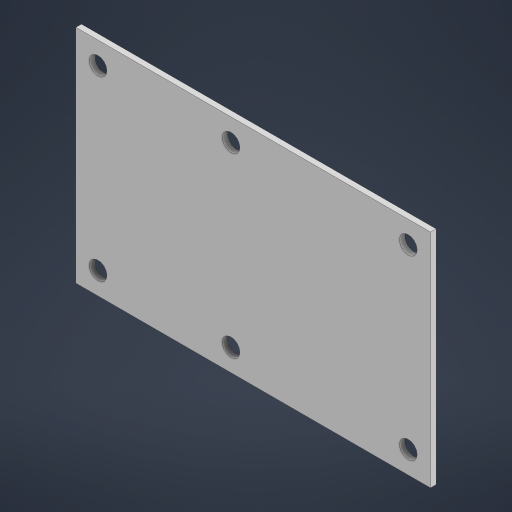
# Autodesk Inventor part: kickPlate
Saved by Autodesk Inventor 2023.4 (Build 274418000, 418)
## iProperties
Created: 2024-01-28
Part Number: kickPlate
Material: Generic
Document SubType Name: Modeling
Designer: Meer
Density: 1 g/cm^3
Appearance: Default
Author: Meer
Autodesk Inventor part; units mm, degrees
ref_plane "YZ Plane" through (0, 0, 0) normal (1, 0, 0) x (0, 1, 0)
ref_plane "XZ Plane" through (0, 0, 0) normal (0, 1, 0) x (-1, 0, 0)
ref_plane "XY Plane" through (0, 0, 0) normal (0, 0, 1) x (1, 0, 0)
sketch "Sketch1" plane through (0, 0, 0) normal (0, 0, 1) x (1, 0, 0)
  line L0 (0, 0) -> (101.6, 0)
  line L1 (101.6, 0) -> (101.6, 63.5)
  line L2 (101.6, 63.5) -> (0, 63.5)
  line L3 (0, 63.5) -> (0, 0)
  line L4 (7.1778, 63.5) -> (7.1778, 57.15)
  line L5 (0, 57.15) -> (6.35, 57.15)
  line L6 (6.35, 57.15) -> (44.45, 57.15)
  line L7 (44.45, 57.15) -> (95.25, 57.15)
  circle A0 centre (44.45, 57.15) radius 2.54
  circle A1 centre (95.25, 57.15) radius 2.54
  circle A2 centre (6.35, 57.15) radius 2.54
  line L8 (6.35, 0) -> (6.35, 6.35)
  line L9 (0, 6.35) -> (6.35, 6.35)
  line L10 (6.35, 6.35) -> (44.45, 6.35)
  line L11 (44.45, 6.35) -> (69.85, 6.35)
  line L12 (69.85, 6.35) -> (95.25, 6.35)
  circle A3 centre (6.35, 6.35) radius 2.54
  circle A4 centre (44.45, 6.35) radius 2.54
  circle A5 centre (95.25, 6.35) radius 2.54
  dimension "d0" = 101.6
  dimension "d1" = 63.5
  dimension "d2" = 6.35
  dimension "d3" = 6.35
  dimension "d5" = 38.1
  dimension "d6" = 50.8
  dimension "d7" = 5.08
  dimension "d8" = 5.08
  dimension "d9" = 5.08
  dimension "d12" = 6.35
  dimension "d13" = 6.35
  dimension "d14" = 38.1
  dimension "d15" = 25.4
  dimension "d16" = 25.4
  dimension "d17" = 5.08
  dimension "d18" = 5.08
  dimension "d19" = 5.08
  constraints: 26 end point, 8 point on line, 7 coincident, 6 centre point, 4 perpendicular, 3 parallel, 2 horizontal
  measures "d0" distance of L2.end L1.end
  measures "d1" distance of L1.end L0.end
  measures "d2" distance of L4.start L4.end
  measures "d3" distance of L5.start L5.end
  measures "d5" distance of L6.start L6.end
  measures "d6" distance of L6.end L7.end
  measures "d7" diameter of A0
  measures "d8" diameter of A1
  measures "d9" diameter of A2
  measures "d12" distance of L8.start L8.end
  measures "d13" distance of L9.start L8.end
  measures "d14" distance of L8.end L10.end
  measures "d15" distance of L10.end L11.end
  measures "d16" distance of L11.end L12.end
  measures "d17" diameter of A3
  measures "d18" diameter of A4
  measures "d19" diameter of A5
extrude "Extrusion1" add sketch "Sketch1" along normal blind 1.5875 contours L3 L9 A3 L8 L0 | L8 A3 L9 L3 L5 A2 L4 L2 L1 L0 | L3 L2 L4 A2 L5
body "Solid1"
